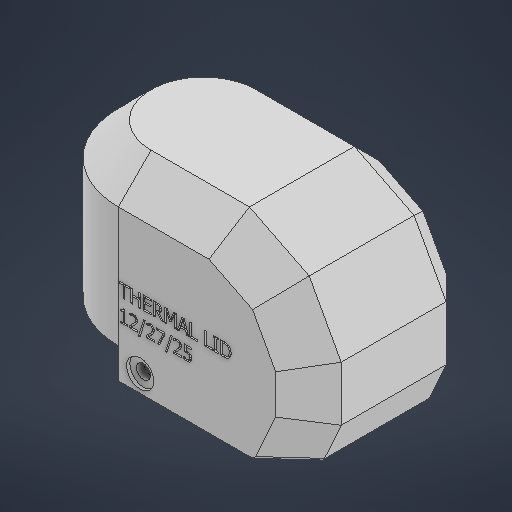
# Autodesk Inventor part: Thermal Lid
Saved by Autodesk Inventor 2026.2 (Build 302298000, 298)
## iProperties
Created: 2025-12-29
Part Number: Thermal Lid
Material: Generic
Document SubType Name: Modeling
Designer: mumin
Density: 1 g/cm^3
Appearance: Default
Author: mumin
Autodesk Inventor part; units mm, degrees
ref_plane "YZ Plane" through (0, 0, 0) normal (1, 0, 0) x (0, 1, 0)
ref_plane "XZ Plane" through (0, 0, 0) normal (0, 1, 0) x (-1, 0, 0)
ref_plane "XY Plane" through (0, 0, 0) normal (0, 0, 1) x (1, 0, 0)
sketch "Sketch1" plane through (0, 0, 0) normal (0, 0, 1) x (1, 0, 0)
  line L0 (0, 0) -> (0, 70)
  line L1 (0, 70) -> (84, 70)
  line L2 (-25.2, 0) -> (151.2, 0) projected
  line L3 (0, 0) -> (100, 0)
  line L4 (126, 4.4656) -> (117.7308, -13.9)
  line L5 (84, 70) -> (111.3558, 56.3184)
  line L6 (111.3558, 56.3184) -> (126, 29.4656)
  line L7 (126, 29.4656) -> (126, 4.4656)
  line L8 (39, 0) -> (39, -13.9)
  line L9 (39, -13.9) -> (117.7308, -13.9)
  point P0 (123.9893, 0)
  dimension "d0" = 70
  dimension "d1" = 84
  dimension "d2" = 42
  dimension "d36" = 100
  dimension "d37" = 65.76
  dimension "d41" = 13.9
  dimension "d42" = 39
  constraints: 18 end point, 3 perpendicular, 2 vertical, 1 collinear, 1 equal length, 1 point on line
  measures "d0" distance of L0.start L0.end
  measures "d1" distance of L0.end L1.end
  measures "d2" horizontal distance of L1.end L4.start
  measures "d36" distance from line of L0 L3.end
  measures "d37" angle of L4 L2
  measures "d41" distance of L8.start L8.end
  measures "d42" distance from line of L8 L0.start
extrude "Bilateral Extrude" add sketch "Sketch1" along normal mid plane 78
sketch "Sketch2" plane through (0, 70, -39) normal (0, 1, 0) x (1, 0, 0)
  line L0 (0, -39) -> (126, -39)
  line L1 (126, 0) -> (126, -78) projected
  line L2 (84, -78) -> (0, -78) projected
  arc A0 (39, 0) -> (39, -78) centre (39, -39) ccw
  line L3 (39, -39) -> (39, 0) construction
  line L4 (39, -39) -> (39, -78) construction
  line L5 (0, 0) -> (0, -78) projected
  line L6 (39, 0) -> (0, 0)
  line L7 (0, -78) -> (39, -78)
  dimension "d6" = 180
  constraints: 10 end point, 2 perpendicular, 2 point on circle, 2 point on line, 2 tangent, 1 centre point, 1 collinear, 1 midpoint
  measures "d6" angle of L3 L4
extrude "Rounded Front" cut sketch "Sketch2" against normal through all
shell "Shell1" thickness 5 removed faces 3 at (28.8362, 0, -8.1054) at (39, -4.6333, 13) at (65.2436, -13.9, -13)
chamfer "Inside Chamfer" distance 12 angle 45 11 edges at (60.9097, 65, 34) (5, 65, 0) (60.9097, 65, -34) (95.2681, 58.7739, 34) (114.3584, 40.3694, 34) (121, 16.8651, 34) (95.2681, 58.7739, -34) (114.3584, 40.3694, -34) (121, 16.8651, -34) (116.6236, -4.1803, -34) (116.6236, -4.1803, 34)
chamfer "Outside Chamfer" distance 15 angle 45 11 edges at (61.5, 70, 39) (0, 70, 0) (61.5, 70, -39) (97.6779, 63.1592, 39) (118.6779, 42.892, 39) (126, 16.9656, 39) (121.8654, -4.7172, 39) (97.6779, 63.1592, -39) (118.6779, 42.892, -39) (126, 16.9656, -39) (121.8654, -4.7172, -39)
sketch "Sketch6" plane through (0, 0, 39) normal (0, 0, 1) x (1, 0, 0)
  line L0 (39.1286, 25.8223) -> (99.692, 25.8223) construction
  line L1 (99.692, 25.8223) -> (99.692, 6.0243) construction
  line L2 (99.692, 6.0243) -> (39.1286, 6.0243) construction
  line L3 (39.1286, 6.0243) -> (39.1286, 25.8223) construction
  line L4 (41.1702, 19.7223) -> (41.1702, 25.1006)
  line L5 (41.1702, 25.1006) -> (39.1237, 25.1006)
  line L6 (39.1237, 25.1006) -> (39.1237, 25.8223)
  line L7 (39.1237, 25.8223) -> (44.0274, 25.8223)
  line L8 (44.0274, 25.8223) -> (44.0274, 25.1006)
  line L9 (44.0274, 25.1006) -> (41.9809, 25.1006)
  line L10 (41.9809, 25.1006) -> (41.9809, 19.7223)
  line L11 (41.9809, 19.7223) -> (41.1702, 19.7223)
  line L12 (49.0745, 19.7223) -> (48.2638, 19.7223)
  line L13 (48.2638, 19.7223) -> (48.2638, 22.708)
  line L14 (48.2638, 22.708) -> (45.456, 22.708)
  line L15 (45.456, 22.708) -> (45.456, 19.7223)
  line L16 (45.456, 19.7223) -> (44.6453, 19.7223)
  line L17 (44.6453, 19.7223) -> (44.6453, 25.8223)
  line L18 (44.6453, 25.8223) -> (45.456, 25.8223)
  line L19 (45.456, 25.8223) -> (45.456, 23.4298)
  line L20 (45.456, 23.4298) -> (48.2638, 23.4298)
  line L21 (48.2638, 23.4298) -> (48.2638, 25.8223)
  line L22 (48.2638, 25.8223) -> (49.0745, 25.8223)
  line L23 (49.0745, 25.8223) -> (49.0745, 19.7223)
  line L24 (50.3103, 19.7223) -> (50.3103, 25.8223)
  line L25 (50.3103, 25.8223) -> (54.1265, 25.8223)
  line L26 (54.1265, 25.8223) -> (54.1265, 25.1006)
  line L27 (54.1265, 25.1006) -> (51.121, 25.1006)
  line L28 (51.121, 25.1006) -> (51.121, 23.4298)
  line L29 (51.121, 23.4298) -> (53.9238, 23.4298)
  line L30 (53.9238, 23.4298) -> (53.9238, 22.708)
  line L31 (53.9238, 22.708) -> (51.121, 22.708)
  line L32 (51.121, 22.708) -> (51.121, 20.444)
  line L33 (51.121, 20.444) -> (54.1265, 20.444)
  line L34 (54.1265, 20.444) -> (54.1265, 19.7223)
  line L35 (54.1265, 19.7223) -> (50.3103, 19.7223)
  line L36 (59.7371, 19.7223) -> (58.6842, 19.7223)
  line L37 (58.6842, 19.7223) -> (56.7563, 22.1495)
  line L38 (56.7563, 22.1495) -> (55.827, 22.1495)
  line L39 (55.827, 22.1495) -> (55.827, 19.7223)
  line L40 (55.827, 19.7223) -> (55.0163, 19.7223)
  line L41 (55.0163, 19.7223) -> (55.0163, 25.8223)
  line L42 (55.0163, 25.8223) -> (56.5882, 25.8223)
  spline S0 degree 2 poles (56.5882, 25.8223) (57.1122, 25.8223) (57.8191, 25.7086) (58.1404, 25.501) knots 0 0 0 1 2 2 2
  spline S1 degree 2 poles (58.1404, 25.501) (58.4617, 25.2934) (58.8325, 24.6458) (58.8325, 24.1663) knots 0 0 0 1 2 2 2
  spline S2 degree 2 poles (58.8325, 24.1663) (58.8325, 23.499) (58.1503, 22.5943) (57.567, 22.3768) knots 0 0 0 1 2 2 2
  line L43 (57.567, 22.3768) -> (59.7371, 19.7223)
  spline S3 degree 2 poles (57.9872, 24.102) (57.9872, 24.369) (57.7993, 24.7793) (57.6016, 24.9127) knots 0 0 0 1 2 2 2
  spline S4 degree 2 poles (57.6016, 24.9127) (57.4286, 25.0264) (56.9689, 25.1204) (56.6327, 25.1204) knots 0 0 0 1 2 2 2
  line L44 (56.6327, 25.1204) -> (55.827, 25.1204)
  line L45 (55.827, 25.1204) -> (55.827, 22.8267)
  line L46 (55.827, 22.8267) -> (56.5388, 22.8267)
  spline S5 degree 2 poles (56.5388, 22.8267) (56.8898, 22.8267) (57.4484, 22.9503) (57.6412, 23.143) knots 0 0 0 1 2 2 2
  spline S6 degree 2 poles (57.6412, 23.143) (57.8191, 23.3111) (57.9872, 23.7857) (57.9872, 24.102) knots 0 0 0 1 2 2 2
  line L47 (65.4515, 19.7223) -> (64.6408, 19.7223)
  line L48 (64.6408, 19.7223) -> (64.6408, 24.977)
  line L49 (64.6408, 24.977) -> (63.0491, 21.403)
  line L50 (63.0491, 21.403) -> (62.5548, 21.403)
  line L51 (62.5548, 21.403) -> (60.9779, 24.977)
  line L52 (60.9779, 24.977) -> (60.9779, 19.7223)
  line L53 (60.9779, 19.7223) -> (60.2215, 19.7223)
  line L54 (60.2215, 19.7223) -> (60.2215, 25.8223)
  line L55 (60.2215, 25.8223) -> (61.3288, 25.8223)
  line L56 (61.3288, 25.8223) -> (62.8514, 22.4263)
  line L57 (62.8514, 22.4263) -> (64.3245, 25.8223)
  line L58 (64.3245, 25.8223) -> (65.4515, 25.8223)
  line L59 (65.4515, 25.8223) -> (65.4515, 19.7223)
  line L60 (66.0299, 19.7223) -> (68.0863, 25.8223)
  line L61 (68.0863, 25.8223) -> (69.0848, 25.8223)
  line L62 (69.0848, 25.8223) -> (71.1412, 19.7223)
  line L63 (71.1412, 19.7223) -> (70.2861, 19.7223)
  line L64 (70.2861, 19.7223) -> (69.7324, 21.4277)
  line L65 (69.7324, 21.4277) -> (67.4041, 21.4277)
  line L66 (67.4041, 21.4277) -> (66.8505, 19.7223)
  line L67 (66.8505, 19.7223) -> (66.0299, 19.7223)
  line L68 (69.51, 22.1198) -> (68.5658, 24.9918)
  line L69 (68.5658, 24.9918) -> (67.6266, 22.1198)
  line L70 (67.6266, 22.1198) -> (69.51, 22.1198)
  line L71 (75.254, 19.7223) -> (71.7196, 19.7223)
  line L72 (71.7196, 19.7223) -> (71.7196, 25.8223)
  line L73 (71.7196, 25.8223) -> (72.5303, 25.8223)
  line L74 (72.5303, 25.8223) -> (72.5303, 20.444)
  line L75 (72.5303, 20.444) -> (75.254, 20.444)
  line L76 (75.254, 20.444) -> (75.254, 19.7223)
  line L77 (82.0461, 19.7223) -> (78.5117, 19.7223)
  line L78 (78.5117, 19.7223) -> (78.5117, 25.8223)
  line L79 (78.5117, 25.8223) -> (79.3224, 25.8223)
  line L80 (79.3224, 25.8223) -> (79.3224, 20.444)
  line L81 (79.3224, 20.444) -> (82.0461, 20.444)
  line L82 (82.0461, 20.444) -> (82.0461, 19.7223)
  line L83 (84.8094, 19.7223) -> (82.4465, 19.7223)
  line L84 (82.4465, 19.7223) -> (82.4465, 20.3452)
  line L85 (82.4465, 20.3452) -> (83.2226, 20.3452)
  line L86 (83.2226, 20.3452) -> (83.2226, 25.1995)
  line L87 (83.2226, 25.1995) -> (82.4465, 25.1995)
  line L88 (82.4465, 25.1995) -> (82.4465, 25.8223)
  line L89 (82.4465, 25.8223) -> (84.8094, 25.8223)
  line L90 (84.8094, 25.8223) -> (84.8094, 25.1995)
  line L91 (84.8094, 25.1995) -> (84.0333, 25.1995)
  line L92 (84.0333, 25.1995) -> (84.0333, 20.3452)
  line L93 (84.0333, 20.3452) -> (84.8094, 20.3452)
  line L94 (84.8094, 20.3452) -> (84.8094, 19.7223)
  spline S7 degree 2 poles (90.6227, 22.7674) (90.6227, 21.9319) (89.9455, 20.5874) (89.377, 20.2117) knots 0 0 0 1 2 2 2
  spline S8 degree 2 poles (89.377, 20.2117) (88.9123, 19.92) (87.9583, 19.7223) (87.2168, 19.7223) knots 0 0 0 1 2 2 2
  line L95 (87.2168, 19.7223) -> (85.8129, 19.7223)
  line L96 (85.8129, 19.7223) -> (85.8129, 25.8223)
  line L97 (85.8129, 25.8223) -> (87.2019, 25.8223)
  spline S9 degree 2 poles (87.2019, 25.8223) (88.0621, 25.8223) (89.0408, 25.5653) (89.3869, 25.3379) knots 0 0 0 1 2 2 2
  spline S10 degree 2 poles (89.3869, 25.3379) (89.9751, 24.9473) (90.6227, 23.6571) (90.6227, 22.7674) knots 0 0 0 1 2 2 2
  spline S11 degree 2 poles (89.7774, 22.7772) (89.7774, 23.4792) (89.3127, 24.4728) (88.853, 24.7546) knots 0 0 0 1 2 2 2
  spline S12 degree 2 poles (88.853, 24.7546) (88.5267, 24.9473) (87.7902, 25.1204) (87.2415, 25.1204) knots 0 0 0 1 2 2 2
  line L98 (87.2415, 25.1204) -> (86.6236, 25.1204)
  line L99 (86.6236, 25.1204) -> (86.6236, 20.4242)
  line L100 (86.6236, 20.4242) -> (87.2415, 20.4242)
  spline S13 degree 2 poles (87.2415, 20.4242) (87.7803, 20.4242) (88.5959, 20.5973) (88.9271, 20.8296) knots 0 0 0 1 2 2 2
  spline S14 degree 2 poles (88.9271, 20.8296) (89.3523, 21.1163) (89.7774, 22.0654) (89.7774, 22.7772) knots 0 0 0 1 2 2 2
  line L101 (43.0288, 9.6788) -> (40.053, 9.6788)
  line L102 (40.053, 9.6788) -> (40.053, 10.3017)
  line L103 (40.053, 10.3017) -> (41.1603, 10.3017)
  line L104 (41.1603, 10.3017) -> (41.1603, 14.3898)
  line L105 (41.1603, 14.3898) -> (40.053, 14.3898)
  line L106 (40.053, 14.3898) -> (40.053, 14.9483)
  spline S15 degree 2 poles (40.053, 14.9483) (40.6808, 14.9483) (41.274, 15.3043) (41.3135, 15.7986) knots 0 0 0 1 2 2 2
  line L107 (41.3135, 15.7986) -> (41.9463, 15.7986)
  line L108 (41.9463, 15.7986) -> (41.9463, 10.3017)
  line L109 (41.9463, 10.3017) -> (43.0288, 10.3017)
  line L110 (43.0288, 10.3017) -> (43.0288, 9.6788)
  line L111 (47.9128, 9.6788) -> (44.151, 9.6788)
  line L112 (44.151, 9.6788) -> (44.151, 10.5439)
  spline S16 degree 2 poles (44.151, 10.5439) (44.5563, 10.9245) (45.278, 11.6314) (45.6241, 12.012) knots 0 0 0 1 2 2 2
  spline S17 degree 2 poles (45.6241, 12.012) (46.3211, 12.7782) (46.8302, 13.6977) (46.8302, 14.1871) knots 0 0 0 1 2 2 2
  spline S18 degree 2 poles (46.8302, 14.1871) (46.8302, 14.4441) (46.672, 14.8297) (46.5287, 14.9533) knots 0 0 0 1 2 2 2
  spline S19 degree 2 poles (46.5287, 14.9533) (46.3853, 15.0769) (46.0096, 15.2005) (45.7822, 15.2005) knots 0 0 0 1 2 2 2
  spline S20 degree 2 poles (45.7822, 15.2005) (45.5647, 15.2005) (45.1198, 15.0917) (44.9172, 15.0077) knots 0 0 0 1 2 2 2
  spline S21 degree 2 poles (44.9172, 15.0077) (44.7442, 14.9385) (44.4228, 14.7407) (44.324, 14.6715) knots 0 0 0 1 2 2 2
  line L113 (44.324, 14.6715) -> (44.2795, 14.6715)
  line L114 (44.2795, 14.6715) -> (44.2795, 15.5415)
  spline S22 degree 2 poles (44.2795, 15.5415) (44.5316, 15.6651) (45.4362, 15.9073) (45.8416, 15.9073) knots 0 0 0 1 2 2 2
  spline S23 degree 2 poles (45.8416, 15.9073) (46.6968, 15.9073) (47.6607, 15.0027) (47.6607, 14.2316) knots 0 0 0 1 2 2 2
  spline S24 degree 2 poles (47.6607, 14.2316) (47.6607, 13.8707) (47.4926, 13.2676) (47.3443, 13.0106) knots 0 0 0 1 2 2 2
  spline S25 degree 2 poles (47.3443, 13.0106) (47.196, 12.7436) (46.766, 12.2197) (46.5287, 11.9675) knots 0 0 0 1 2 2 2
  spline S26 degree 2 poles (46.5287, 11.9675) (46.1431, 11.5474) (45.1989, 10.6477) (44.9172, 10.3857) knots 0 0 0 1 2 2 2
  line L115 (44.9172, 10.3857) -> (47.9128, 10.3857)
  line L116 (47.9128, 10.3857) -> (47.9128, 9.6788)
  line L117 (51.2643, 16.0507) -> (48.8767, 8.354)
  line L118 (48.8767, 8.354) -> (48.1847, 8.354)
  line L119 (48.1847, 8.354) -> (50.5624, 16.0507)
  line L120 (50.5624, 16.0507) -> (51.2643, 16.0507)
  line L121 (55.6985, 9.6788) -> (51.9366, 9.6788)
  line L122 (51.9366, 9.6788) -> (51.9366, 10.5439)
  spline S27 degree 2 poles (51.9366, 10.5439) (52.342, 10.9245) (53.0637, 11.6314) (53.4097, 12.012) knots 0 0 0 1 2 2 2
  spline S28 degree 2 poles (53.4097, 12.012) (54.1067, 12.7782) (54.6159, 13.6977) (54.6159, 14.1871) knots 0 0 0 1 2 2 2
  spline S29 degree 2 poles (54.6159, 14.1871) (54.6159, 14.4441) (54.4577, 14.8297) (54.3143, 14.9533) knots 0 0 0 1 2 2 2
  spline S30 degree 2 poles (54.3143, 14.9533) (54.171, 15.0769) (53.7953, 15.2005) (53.5679, 15.2005) knots 0 0 0 1 2 2 2
  spline S31 degree 2 poles (53.5679, 15.2005) (53.3504, 15.2005) (52.9055, 15.0917) (52.7028, 15.0077) knots 0 0 0 1 2 2 2
  spline S32 degree 2 poles (52.7028, 15.0077) (52.5298, 14.9385) (52.2085, 14.7407) (52.1096, 14.6715) knots 0 0 0 1 2 2 2
  line L123 (52.1096, 14.6715) -> (52.0651, 14.6715)
  line L124 (52.0651, 14.6715) -> (52.0651, 15.5415)
  spline S33 degree 2 poles (52.0651, 15.5415) (52.3173, 15.6651) (53.2219, 15.9073) (53.6272, 15.9073) knots 0 0 0 1 2 2 2
  spline S34 degree 2 poles (53.6272, 15.9073) (54.4824, 15.9073) (55.4463, 15.0027) (55.4463, 14.2316) knots 0 0 0 1 2 2 2
  spline S35 degree 2 poles (55.4463, 14.2316) (55.4463, 13.8707) (55.2783, 13.2676) (55.13, 13.0106) knots 0 0 0 1 2 2 2
  spline S36 degree 2 poles (55.13, 13.0106) (54.9817, 12.7436) (54.5516, 12.2197) (54.3143, 11.9675) knots 0 0 0 1 2 2 2
  spline S37 degree 2 poles (54.3143, 11.9675) (53.9288, 11.5474) (52.9846, 10.6477) (52.7028, 10.3857) knots 0 0 0 1 2 2 2
  line L125 (52.7028, 10.3857) -> (55.6985, 10.3857)
  line L126 (55.6985, 10.3857) -> (55.6985, 9.6788)
  line L127 (60.3451, 14.8643) -> (57.7054, 9.6788)
  line L128 (57.7054, 9.6788) -> (56.8354, 9.6788)
  line L129 (56.8354, 9.6788) -> (59.6234, 15.062)
  line L130 (59.6234, 15.062) -> (56.4745, 15.062)
  line L131 (56.4745, 15.062) -> (56.4745, 15.7788)
  line L132 (56.4745, 15.7788) -> (60.3451, 15.7788)
  line L133 (60.3451, 15.7788) -> (60.3451, 14.8643)
  line L134 (63.6275, 16.0507) -> (61.2399, 8.354)
  line L135 (61.2399, 8.354) -> (60.5478, 8.354)
  line L136 (60.5478, 8.354) -> (62.9255, 16.0507)
  line L137 (62.9255, 16.0507) -> (63.6275, 16.0507)
  line L138 (68.0616, 9.6788) -> (64.2997, 9.6788)
  line L139 (64.2997, 9.6788) -> (64.2997, 10.5439)
  spline S38 degree 2 poles (64.2997, 10.5439) (64.7051, 10.9245) (65.4268, 11.6314) (65.7728, 12.012) knots 0 0 0 1 2 2 2
  spline S39 degree 2 poles (65.7728, 12.012) (66.4698, 12.7782) (66.979, 13.6977) (66.979, 14.1871) knots 0 0 0 1 2 2 2
  spline S40 degree 2 poles (66.979, 14.1871) (66.979, 14.4441) (66.8208, 14.8297) (66.6775, 14.9533) knots 0 0 0 1 2 2 2
  spline S41 degree 2 poles (66.6775, 14.9533) (66.5341, 15.0769) (66.1584, 15.2005) (65.931, 15.2005) knots 0 0 0 1 2 2 2
  spline S42 degree 2 poles (65.931, 15.2005) (65.7135, 15.2005) (65.2686, 15.0917) (65.066, 15.0077) knots 0 0 0 1 2 2 2
  spline S43 degree 2 poles (65.066, 15.0077) (64.8929, 14.9385) (64.5716, 14.7407) (64.4728, 14.6715) knots 0 0 0 1 2 2 2
  line L140 (64.4728, 14.6715) -> (64.4283, 14.6715)
  line L141 (64.4283, 14.6715) -> (64.4283, 15.5415)
  spline S44 degree 2 poles (64.4283, 15.5415) (64.6804, 15.6651) (65.585, 15.9073) (65.9903, 15.9073) knots 0 0 0 1 2 2 2
  spline S45 degree 2 poles (65.9903, 15.9073) (66.8455, 15.9073) (67.8095, 15.0027) (67.8095, 14.2316) knots 0 0 0 1 2 2 2
  spline S46 degree 2 poles (67.8095, 14.2316) (67.8095, 13.8707) (67.6414, 13.2676) (67.4931, 13.0106) knots 0 0 0 1 2 2 2
  spline S47 degree 2 poles (67.4931, 13.0106) (67.3448, 12.7436) (66.9147, 12.2197) (66.6775, 11.9675) knots 0 0 0 1 2 2 2
  spline S48 degree 2 poles (66.6775, 11.9675) (66.2919, 11.5474) (65.3477, 10.6477) (65.066, 10.3857) knots 0 0 0 1 2 2 2
  line L142 (65.066, 10.3857) -> (68.0616, 10.3857)
  line L143 (68.0616, 10.3857) -> (68.0616, 9.6788)
  spline S49 degree 2 poles (72.5748, 11.6166) (72.5748, 11.1766) (72.293, 10.4252) (72.036, 10.1484) knots 0 0 0 1 2 2 2
  spline S50 degree 2 poles (72.036, 10.1484) (71.7789, 9.8716) (71.0127, 9.5503) (70.5382, 9.5503) knots 0 0 0 1 2 2 2
  spline S51 degree 2 poles (70.5382, 9.5503) (70.1032, 9.5503) (69.2529, 9.7431) (68.9415, 9.8963) knots 0 0 0 1 2 2 2
  line L144 (68.9415, 9.8963) -> (68.9415, 10.7614)
  line L145 (68.9415, 10.7614) -> (69.0008, 10.7614)
  spline S52 degree 2 poles (69.0008, 10.7614) (69.0947, 10.6922) (69.4457, 10.5142) (69.6583, 10.4351) knots 0 0 0 1 2 2 2
  spline S53 degree 2 poles (69.6583, 10.4351) (69.9005, 10.3511) (70.3009, 10.2572) (70.553, 10.2572) knots 0 0 0 1 2 2 2
  spline S54 degree 2 poles (70.553, 10.2572) (70.8002, 10.2572) (71.2648, 10.4351) (71.4329, 10.6279) knots 0 0 0 1 2 2 2
  spline S55 degree 2 poles (71.4329, 10.6279) (71.5861, 10.8108) (71.7443, 11.2953) (71.7443, 11.6215) knots 0 0 0 1 2 2 2
  spline S56 degree 2 poles (71.7443, 11.6215) (71.7443, 11.9478) (71.5664, 12.363) (71.3983, 12.5014) knots 0 0 0 1 2 2 2
  spline S57 degree 2 poles (71.3983, 12.5014) (71.2253, 12.6547) (70.7112, 12.7832) (70.3997, 12.7832) knots 0 0 0 1 2 2 2
  spline S58 degree 2 poles (70.3997, 12.7832) (70.0636, 12.7832) (69.3963, 12.6794) (69.1936, 12.6349) knots 0 0 0 1 2 2 2
  line L146 (69.1936, 12.6349) -> (69.1936, 15.7788)
  line L147 (69.1936, 15.7788) -> (72.5402, 15.7788)
  line L148 (72.5402, 15.7788) -> (72.5402, 15.062)
  line L149 (72.5402, 15.062) -> (69.9796, 15.062)
  line L150 (69.9796, 15.062) -> (69.9796, 13.4357)
  spline S59 degree 2 poles (69.9796, 13.4357) (70.1279, 13.4555) (70.4146, 13.4703) (70.5332, 13.4703) knots 0 0 0 1 2 2 2
  spline S60 degree 2 poles (70.5332, 13.4703) (71.0028, 13.4703) (71.6504, 13.3171) (71.947, 13.0897) knots 0 0 0 1 2 2 2
  spline S61 degree 2 poles (71.947, 13.0897) (72.2485, 12.8623) (72.5748, 12.1702) (72.5748, 11.6166) knots 0 0 0 1 2 2 2
  point P0 (0, 0)
  constraints: 2 other
emboss "LABEL" sketch "Sketch6" operation cut depth 1 direction (0, 0, -1)
fillet "Fillet2" radius 2 6 edges at (105.6671, -13.9, 28) (112.2473, -13.9, 0) (105.6671, -13.9, -28) (109.5056, -13.9, 31.5) (117.7308, -13.9, 0) (109.5056, -13.9, -31.5)
sketch "Sketch7" plane through (0, 0, 39) normal (0, 0, 1) x (1, 0, 0)
  line L0 (39, 0) -> (39, -13.9) projected
  point P0 (0, 0)
  point P1 (49, -6)
  dimension "d51" = 10
  dimension "d52" = 6
  measures "d51" distance from line of L0 point (49, -6)
  measures "d52" vertical distance of L0.start point (49, -6)
hole "Hole2" at (49, -6, 39) direction (0, 0, -1) diameter 6.5 end up to face face through (75.9953, 20.3721, 34) facing (0, 0, -1) counterbore diameter 12.5 counterbore depth 1.5
mirror "Mirror2" about plane through (0, 0, 0) normal (0, 0, 1) of "Hole2"
body "Solid1"
